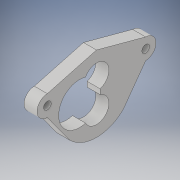
# Autodesk Inventor part: MotorFixedPositionMount
Saved by Autodesk Inventor 2017 (Build 210142000, 142)
## iProperties
Created: 2017-08-12
Part Number: MotorFixedPositionMount
Material: Generic
Document SubType Name: Modeling
Designer: User
Density: 1 g/cm^3
Appearance: Default
Author: User
Autodesk Inventor part; units mm, degrees
ref_plane "YZ Plane" through (0, 0, 0) normal (1, 0, 0) x (0, 1, 0)
ref_plane "XZ Plane" through (0, 0, 0) normal (0, 1, 0) x (-1, 0, 0)
ref_plane "XY Plane" through (0, 0, 0) normal (0, 0, 1) x (1, 0, 0)
sketch "Sketch1" plane through (0, 0, 0) normal (1, 0, 0) x (0, 1, 0)
  arc A0 (1.2261, -1.7474) -> (9.7245, 5.3822) centre (7, 0) ccw
  arc A1 (-9.7245, 5.3822) -> (-1.2261, -1.7474) centre (-7, 0) ccw
  arc A2 (9.7245, 5.3822) -> (-9.7245, 5.3822) centre (0, 8.3439) ccw
  arc A3 (-1.2261, -1.7474) -> (1.2261, -1.7474) centre (0, 8.3439) ccw
  circle A4 centre (7.0104, 24.0085) radius 1.8542
  circle A5 centre (7.0104, -23.9975) radius 1.8542
  arc A6 (12.0396, 24.0085) -> (1.9812, 24.0085) centre (7.0104, 24.0085) ccw
  arc A7 (1.9812, -23.9975) -> (12.0396, -23.9975) centre (7.0104, -23.9975) ccw
  line L0 (12.0396, 24.0085) -> (18.5, 0.0055)
  line L1 (12.0396, -23.9975) -> (18.5, 0.0055)
  line L2 (1.9812, 24.0085) -> (-13.0815, 13.087)
  line L3 (-13.0815, -13.0759) -> (1.9812, -23.9975)
  arc A8 (0.4193, 18.5008) -> (-0.4193, 18.5008) centre (0, 0.0055) ccw
  arc A9 (-13.0815, 13.087) -> (-13.0815, -13.0759) centre (0, 0.0055) ccw
  point P0 (0, 0)
  dimension "d0" = 12.065
  dimension "d1" = 7
  dimension "d2" = 12.065
  dimension "d3" = 7
  dimension "d7" = 8.3439
  dimension "d8" = 3.7084
  dimension "d11" = 3.7084
  dimension "d14" = 10.0584
  dimension "d15" = 10.0584
  dimension "d26" = 10.1655
  constraints: 18 point on circle, 10 centre point, 8 end point, 2 coincident
  measures "d0" diameter of A0
  measures "d1" distance of point (0, 0) A0.centre
  measures "d2" diameter of A1
  measures "d3" distance of A1.centre point (0, 0)
  measures "d7" distance of point (0, 0) A2.centre
  measures "d8" diameter of A4
  measures "d11" diameter of A5
  measures "d14" diameter of A6
  measures "d15" diameter of A7
  measures "d26" radius of A2
extrude "Extrusion1" add sketch "Sketch1" along normal blind 6.35
body "Solid1"
